chrismas v0_v5 (Autodesk Fusion 360 design; units mm, degrees)
Autodesk Fusion 360 part; units mm, degrees
sketch "christmas tree" plane through (0, 0, 0) normal (0, 0, 1) x (1, 0, 0)
  line L0 (46, 3) -> (58, 3)
  line L1 (58, 3) -> (58, 34.8153)
  line L2 (46, 35.3486) -> (46, 3)
  line L3 (-4.5818, 19.2349) -> (37.2552, 60.6233)
  line L4 (68.2313, 66.0117) -> (107.184, 26.6368)
  line L5 (-4.5818, 19.2349) -> (46, 34.2237)
  line L6 (58, 34.8153) -> (107.184, 26.6368)
  line L7 (67.9006, 91.943) -> (94.9514, 63.5826)
  line L8 (8.3421, 56.9885) -> (37.2552, 60.6233)
  line L9 (8.3421, 56.9885) -> (44, 91)
  line L10 (68.2313, 66.0117) -> (94.9514, 63.5826)
  line L11 (66.5924, 110.4813) -> (88.365, 85.994)
  line L12 (67.9006, 91.943) -> (88.365, 85.994)
  line L13 (19.0375, 83.8717) -> (44, 91)
  line L14 (19.0375, 83.8717) -> (45.5444, 107.44)
  line L15 (66.5924, 110.4813) -> (79.9118, 107.17)
  line L16 (30.0026, 103.3259) -> (45.5444, 107.44)
  line L17 (30.0026, 103.3259) -> (53.841, 137.6532)
  line L18 (79.9118, 107.17) -> (58.0039, 139.3622)
  line L19 (46.4668, 151.7481) -> (51.8961, 142.7662)
  line L20 (54.9383, 145.3446) -> (46.4668, 151.7481)
  line L21 (43.1882, 136.688) -> (53.4083, 139.0761)
  line L22 (51.8961, 142.7662) -> (43.1882, 136.688)
  line L23 (53.4083, 139.0761) -> (53.841, 137.6532)
  line L24 (58.0039, 139.3622) -> (68.0025, 139.1729)
  line L25 (61.8029, 153.2838) -> (54.9383, 145.3446)
  line L26 (58.3306, 143.2481) -> (61.8029, 153.2838)
  line L27 (68.0025, 139.1729) -> (58.3306, 143.2481)
  point P0 (56.5309, 66.7861)
  constraint horizontal L0
  constraint vertical L1
  constraint vertical L2
  constraint perpendicular L3 L4
  constraint coincident L4 L6.end
  constraint perpendicular L7 L9
  constraint perpendicular L11 L14
  constraint coincident L2 L5.end
extrude "Extrude23" add sketch "christmas tree" along normal blind 0.4
equation "fingerWidth = 10 mm"
equation "length = 80 mm"
equation "thickness = 3.175 mm"
equation "height = 45 mm"
equation "toolDiameter = 2 mm"
equation "boneCenterToHoleBottom = toolDiameter / 2 / sqrt(2) - 0 * kerf" comment "Best: 2.001 -2*kerf, 0.1;;;Best: 2.001 no kerf and 0.1   OLD+6 kerf at 2.001 Diam and .1 mm"
equation "tempLengthPieces = ceil(( ( floor(( length - 2 * thickness ) / fingerWidth) - 2 ) - ( ( floor(( length - 2 * thickness ) / fingerWidth) - 2 ) % 2 - 1 ) ))"
equation "lengthCuts = ceil(tempLengthPieces / 2)"
equation "shoulderToothLength = ( length - fingerWidth * tempLengthPieces ) / 2 - kerf"
equation "depth = 50 mm"
equation "tempDepthPieces = ceil(( ( floor(( depth - 2 * thickness ) / fingerWidth) - 2 ) - ( ( floor(( depth - 2 * thickness ) / fingerWidth) - 2 ) % 2 - 1 ) ))"
equation "depthCuts = ceil(tempDepthPieces / 2)"
equation "shoulderToothDepth = ( depth - fingerWidth * tempDepthPieces ) / 2 - kerf"
equation "tempHeightPieces = ceil(( ( floor(( height - 2 * thickness ) / fingerWidth) - 2 ) - ( ( floor(( height - 2 * thickness ) / fingerWidth) - 2 ) % 2 - 1 ) ))"
equation "heightCuts = ceil(tempHeightPieces / 2)"
equation "sholderToothHeight = ( height - fingerWidth * tempHeightPieces ) / 2 - kerf"
equation "kerf = -0.095 mm"
equation "holeWidth = fingerWidth + 2 * kerf"
equation "shoulderHoleLength = shoulderToothLength + 2 * kerf"
equation "shouderHoleDepth = shoulderToothDepth + 2 * kerf"
equation "shoulderHoleHeight = sholderToothHeight + 2 * kerf"
equation "assembleScrewDiam = 2.1 mm"
equation "assembleScrewDistance = 6 mm"
equation "assembleAvoidCollisionDistance = 1 mm"
equation "coolingHoleDistance = 8 mm"
equation "boneCornerToCenterPack = -3 * kerf"
equation "boneCenterToHoleSide = boneCenterToHoleBottom - boneCornerToCenterPack"
equation "pumpLength = 52 mm"
equation "pumpCircleDiam = 30 mm"
equation "pumpHeight = 34 mm"
equation "sensorWireDistance = 10 mm"
equation "sensorWireDiam = 3.5 mm"
equation "pumpScrewDiam = 3 mm"
equation "pcbMountHoles = 2 mm"
equation "ventDiameter = 3 mm"
equation "platformGrommetMountDiameter = 3.5 mm"
equation "hangerWireDiameter = 2 mm"
equation "topPillowHoleDistance = 22 mm"
equation "extraLineHeight = ( max(-appendix + ( sholderToothHeight - thickness ); 0.001 mm) )"
equation "appendix = fingerWidth - 2 * kerf"
equation "extraLineLength = ( max(-appendix + ( shoulderToothLength ); 0.001 mm) )"
equation "extraLineDepth = ( max(-appendix + ( shoulderToothDepth ); 0.001 mm) )"
